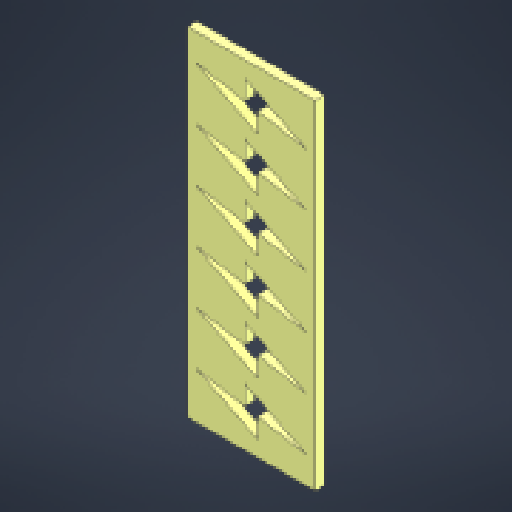
# Autodesk Inventor part: panel
Saved by Autodesk Inventor 2024.3 (Build 283343000, 343)
## iProperties
Created: 2025-08-06
Part Number: panel
Material: Generic
Document SubType Name: Modeling
Designer: giuseppe
Density: 1 g/cm^3
Appearance: Default
Author: giuseppe
Autodesk Inventor part; units mm, degrees
ref_plane "YZ Plane" through (0, 0, 0) normal (1, 0, 0) x (0, 1, 0)
ref_plane "XZ Plane" through (0, 0, 0) normal (0, 1, 0) x (-1, 0, 0)
ref_plane "XY Plane" through (0, 0, 0) normal (0, 0, 1) x (1, 0, 0)
sketch "Sketch1" plane through (0, 0, 0) normal (0, 0, 1) x (1, 0, 0)
  line L0 (20, 36.2675) -> (-20, 36.2675)
  line L1 (-20, 36.2675) -> (-20, -36.2675)
  line L2 (-20, -36.2675) -> (20, -36.2675)
  line L3 (20, -36.2675) -> (20, 36.2675)
  line L4 (17, 6.5024) -> (2, 9.1473)
  line L5 (2, 9.1473) -> (2, 3)
  line L6 (2, 3) -> (-17, 12.4976)
  line L7 (-17, 12.4976) -> (-2, 9.8527)
  line L8 (-2, 9.8527) -> (-2, 16)
  line L9 (-2, 16) -> (17, 6.5024)
  line L10 (-2, 16) -> (2, 16) construction
  line L11 (2, 16) -> (2, 3) construction
  line L12 (2, 3) -> (-2, 3) construction
  line L13 (-2, 3) -> (-2, 16) construction
  point P0 (0, 0)
  point P1 (20, 0)
  point P2 (0, 36.2675)
  point P3 (0, 16)
  dimension "d0" = 40
  dimension "d1" = 4
  dimension "d2" = 3
  dimension "d3" = 80
  dimension "d4" = 13
  dimension "d5" = 3
  constraints: 28 end point, 7 parallel, 3 collinear, 3 midpoint, 2 horizontal, 2 perpendicular, 2 vertical alignment, 1 horizontal alignment
  measures "d0" distance of L0.start L0.end
  measures "d1" distance between parallel lines of L5 L8
  measures "d2" distance from line of L3 L4.start
  measures "d3" angle of L4 L5
  measures "d4" distance of L12.end L8.end
  measures "d5" vertical distance of L5.end point (0, 0)
extrude "Extrusion1" add sketch "Sketch1" along normal blind 10 contours L4 L5 L6 L7 L8 L9
pattern_linear "Rectangular Pattern1" count 6 spacing 16.5 along (0, -1, 0) of "Extrusion1"
sketch "Sketch2" plane through (0, 0, 10) normal (0, 0, 1) x (1, 0, 0)
  line L0 (20, 21) -> (-20, 21)
  line L1 (-20, 21) -> (-20, -84.5)
  line L2 (-20, -84.5) -> (20, -84.5)
  line L3 (20, -84.5) -> (20, 21)
  line L4 (-2, 16) -> (-2, 9.8527) construction
  line L5 (-2, 9.8527) -> (-17, 12.4976) construction
  line L6 (-17, 12.4976) -> (2, 3) construction
  line L7 (2, 3) -> (2, 9.1473) construction
  line L8 (2, 9.1473) -> (17, 6.5024) construction
  line L9 (17, 6.5024) -> (-2, 16) construction
  line L10 (-2, -66.5) -> (-2, -72.6473) construction
  line L11 (-2, -72.6473) -> (-17, -70.0024) construction
  line L12 (-17, -70.0024) -> (2, -79.5) construction
  line L13 (2, -79.5) -> (2, -73.3527) construction
  line L14 (2, -73.3527) -> (17, -75.9976) construction
  line L15 (17, -75.9976) -> (-2, -66.5) construction
  point P0 (0, 0)
  point P1 (0, 21)
  dimension "d11" = 40
  dimension "d12" = 5
  dimension "d13" = 5
  constraints: 8 end point, 2 parallel, 1 horizontal, 1 midpoint, 1 perpendicular, 1 vertical alignment
  measures "d11" distance of L0.start L0.end
  measures "d12" distance from line of L0 L4.start
  measures "d13" distance from line of L12.end L2
extrude "Extrusion2" add sketch "Sketch2" along normal blind 3
sketch "Sketch3" plane through (-2, -72.6473, 0) normal (0, 0, -1) x (-1, 0, 0)
  line L0 (0, 6.1473) -> (0, 0) projected
  line L1 (-19, -3.3502) -> (0, 6.1473) projected
  line L2 (-4, -0.7053) -> (-19, -3.3502) projected
  line L3 (-4, -6.8527) -> (-4, -0.7053) projected
  line L4 (15, 2.6449) -> (-4, -6.8527) projected
  line L5 (0, 0) -> (15, 2.6449) projected
  line L6 (0, 22.6473) -> (0, 16.5) projected
  line L7 (-19, 13.1498) -> (0, 22.6473) projected
  line L8 (-4, 15.7947) -> (-19, 13.1498) projected
  line L9 (-4, 9.6473) -> (-4, 15.7947) projected
  line L10 (15, 19.1449) -> (-4, 9.6473) projected
  line L11 (0, 16.5) -> (15, 19.1449) projected
  line L12 (0, 39.1473) -> (0, 33) projected
  line L13 (-19, 29.6498) -> (0, 39.1473) projected
  line L14 (-4, 32.2947) -> (-19, 29.6498) projected
  line L15 (-4, 26.1473) -> (-4, 32.2947) projected
  line L16 (15, 35.6449) -> (-4, 26.1473) projected
  line L17 (0, 33) -> (15, 35.6449) projected
  line L18 (0, 55.6473) -> (0, 49.5) projected
  line L19 (-19, 46.1498) -> (0, 55.6473) projected
  line L20 (-4, 48.7947) -> (-19, 46.1498) projected
  line L21 (-4, 42.6473) -> (-4, 48.7947) projected
  line L22 (15, 52.1449) -> (-4, 42.6473) projected
  line L23 (0, 49.5) -> (15, 52.1449) projected
  line L24 (0, 72.1473) -> (0, 66) projected
  line L25 (-19, 62.6498) -> (0, 72.1473) projected
  line L26 (-4, 65.2947) -> (-19, 62.6498) projected
  line L27 (-4, 59.1473) -> (-4, 65.2947) projected
  line L28 (15, 68.6449) -> (-4, 59.1473) projected
  line L29 (0, 66) -> (15, 68.6449) projected
  line L30 (0, 88.6473) -> (0, 82.5) projected
  line L31 (-19, 79.1498) -> (0, 88.6473) projected
  line L32 (-4, 81.7947) -> (-19, 79.1498) projected
  line L33 (-4, 75.6473) -> (-4, 81.7947) projected
  line L34 (15, 85.1449) -> (-4, 75.6473) projected
  line L35 (0, 82.5) -> (15, 85.1449) projected
  point P0 (-2, 72.6473)
extrude "Extrusion3" cut sketch "Sketch3" against normal through all
body "Solid1"
